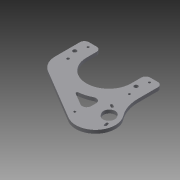
# Autodesk Inventor part: CAD:motor_plate
Saved by Autodesk Inventor 2015 (Build 190159000, 159)
## iProperties
Created: 2015-08-30
Material: Generic
Description: motor mount plate
Document SubType Name: Modeling
Designer: francis
Density: 1 g/cm^3
Appearance: Default
Part Category: insert part category here and press enter to fill value
Author: francis
Autodesk Inventor part; units mm, degrees
ref_plane "YZ Plane" through (0, 0, 0) normal (1, 0, 0) x (0, 1, 0)
ref_plane "XZ Plane" through (0, 0, 0) normal (0, 1, 0) x (-1, 0, 0)
ref_plane "XY Plane" through (0, 0, 0) normal (0, 0, 1) x (1, 0, 0)
sketch "Sketch1" plane through (0, 0, 0) normal (0, 0, 1) x (1, 0, 0)
  circle A0 centre (-18.2965, -47.165) radius 1.2295 construction
  circle A1 centre (-6.0724, -26.0926) radius 1.2295 construction
  circle A2 centre (5.6859, -42.8853) radius 1.2295 construction
  circle A3 centre (-0.1932, -34.489) radius 6 construction
  circle A4 centre (-7.5, -9) radius 1.621 construction
  circle A5 centre (-10.5, 0) radius 2.067 construction
  circle A6 centre (-7.5, 9) radius 1.621 construction
  circle A7 centre (-35, 0) radius 4 construction
  circle A8 centre (-62.5, 9) radius 1.621 construction
  line L0 (-55, -16) -> (-55, 16) construction
  circle A9 centre (-65.5, 0) radius 2.067 construction
  circle A10 centre (-62.5, -9) radius 1.621 construction
  circle A11 centre (-65.5, 0) radius 2.067 construction
  circle A12 centre (-62.5, 9) radius 1.7295 construction
  circle A13 centre (-62.5, -9) radius 1.7295 construction
  line L1 (-70, 13.1624) -> (-55, 13.1624) construction
  line L2 (-70, -13.1624) -> (-70, 13.1624) construction
  line L3 (-55, -13.1624) -> (-70, -13.1624) construction
  line L4 (-55, 13.1624) -> (-55, -13.1624) construction
  circle A14 centre (-10.5, 0) radius 2.067 construction
  circle A15 centre (-7.5, -9) radius 1.621 construction
  circle A16 centre (-7.5, 9) radius 1.621 construction
  line L5 (-15, 13.1624) -> (0, 13.1624) construction
  line L6 (-15, -13.1624) -> (-15, 13.1624) construction
  line L7 (0, -13.1624) -> (-15, -13.1624) construction
  line L8 (0, 13.1624) -> (0, -13.1624) construction
  arc A17 (4.363, -44.1343) -> (4.0127, -42.1709) centre (-18.2965, -47.165) ccw
  arc A18 (7.3366, -43.7366) -> (6.9402, -41.5156) centre (-18.2965, -47.165) ccw
  arc A19 (-5.9734, -27.9093) -> (-7.6985, -26.9086) centre (-18.2965, -47.165) ccw
  arc A20 (-4.3563, -25.3825) -> (-6.3078, -24.2504) centre (-18.2965, -47.165) ccw
  arc A21 (-4.9287, -38.6488) -> (-5.7218, -37.5161) centre (-18.2965, -47.165) ccw
  arc A22 (5.6137, -31.9325) -> (4.1951, -29.9066) centre (-18.2965, -47.165) ccw
  arc A23 (-5.1648, -26.6459) -> (-7.0032, -25.5795) centre (-18.2965, -47.165) ccw construction
  arc A24 (0.3425, -35.2907) -> (-0.7634, -33.7114) centre (-18.2965, -47.165) ccw construction
  arc A25 (5.8498, -43.9354) -> (5.4764, -41.8432) centre (-18.2965, -47.165) ccw construction
  arc A26 (6.9402, -41.5156) -> (4.0127, -42.1709) centre (5.4764, -41.8432) ccw
  arc A27 (4.363, -44.1343) -> (7.3366, -43.7366) centre (5.8498, -43.9354) ccw
  arc A28 (-4.9287, -38.6488) -> (5.6137, -31.9325) centre (0.3425, -35.2907) ccw
  arc A29 (4.1951, -29.9066) -> (-5.7218, -37.5161) centre (-0.7634, -33.7114) ccw
  arc A30 (-5.9734, -27.9093) -> (-4.3563, -25.3825) centre (-5.1648, -26.6459) ccw
  arc A31 (-6.3078, -24.2504) -> (-7.6985, -26.9086) centre (-7.0032, -25.5795) ccw
  circle A32 centre (-18.2965, -47.165) radius 1.5
  circle A33 centre (-7.5, -9) radius 2
  circle A34 centre (-7.5, 9) radius 2
  circle A35 centre (-10.5, 0) radius 2.5
  circle A36 centre (-62.5, 9) radius 2
  circle A37 centre (-65.5, 0) radius 2.5
  circle A38 centre (-62.5, -9) radius 2
  circle A39 centre (-7.3444, -39.4963) radius 17.7 construction
  arc A40 (-16.3879, -54.7116) -> (6.7463, -28.7846) centre (-7.3444, -39.4963) ccw
  arc A41 (0, -8.7624) -> (6.7463, -28.7846) centre (33.0845, -8.7624) ccw
  line L9 (0, -8.7624) -> (0, 9.1624)
  line L10 (-11, 13.1624) -> (-4, 13.1624)
  line L11 (-15, 9.1624) -> (-15, 0)
  line L12 (-55, 0) -> (-55, 9.1624)
  line L13 (-66, 13.1624) -> (-59, 13.1624)
  line L14 (-70, 9.1624) -> (-70, -13.1624)
  arc A42 (-55, 0) -> (-15, 0) centre (-35, 0) ccw
  arc A43 (-66, 13.1624) -> (-70, 9.1624) centre (-66, 9.1624) ccw
  arc A44 (-55, 9.1624) -> (-59, 13.1624) centre (-59, 9.1624) ccw
  arc A45 (-11, 13.1624) -> (-15, 9.1624) centre (-11, 9.1624) ccw
  arc A46 (0, 9.1624) -> (-4, 13.1624) centre (-4, 9.1624) ccw
  line L15 (-61.6755, -27.7942) -> (-16.3879, -54.7116)
  arc A47 (-70, -13.1624) -> (-61.6755, -27.7942) centre (-52.9789, -13.1624) ccw
  arc A48 (-35.0864, -30.8138) -> (-21.0883, -27.4948) centre (-35, 0) ccw
  line L16 (-35.0864, -30.8138) -> (-21.3261, -38.9925)
  line L17 (-15.2824, -31.0639) -> (-15.2824, -35.554)
  arc A49 (-15.2824, -31.0639) -> (-21.0883, -27.4948) centre (-19.2824, -31.0639) ccw
  arc A50 (-21.3261, -38.9925) -> (-15.2824, -35.554) centre (-19.2824, -35.554) ccw
  point P0 (0, 0)
  point P1 (-15.2824, -23.6794)
  dimension "d0" = 3
  dimension "d1" = 5
  dimension "d2" = 5
  dimension "d3" = 5
  dimension "d4" = 12.5
  dimension "d5" = 3
  dimension "d6" = 4
  dimension "d7" = 4
  dimension "d8" = 5
  dimension "d9" = 4
  dimension "d10" = 5
  dimension "d11" = 4
  dimension "d12" = 4
  dimension "d15" = 4
  constraints: 61 point on circle, 33 centre point, 29 tangent, 23 coincident, 20 end point, 10 point on line, 7 equal radius, 4 collinear, 2 midpoint, 1 perpendicular, 1 vertical
  measures "d0" radial gap between concentric circles of A18 A17
  measures "d4" radial gap between concentric circles of A22 A21
  measures "d5" diameter of A32
  measures "d6" diameter of A33
  measures "d7" diameter of A34
  measures "d8" diameter of A35
  measures "d9" diameter of A36
  measures "d10" diameter of A37
  measures "d11" diameter of A38
  measures "d12" radius of A43
  measures "d15" radius of A49
extrude "Extrusion1" add sketch "Sketch1" along normal blind 3
sketch "Sketch2" plane through (0, 0, 3) normal (0, 0, 1) x (1, 0, 0)
  arc A0 (4.1951, -29.9066) -> (-5.7218, -37.5161) centre (-0.7634, -33.7114) ccw projected
  arc A1 (5.6137, -31.9325) -> (4.1951, -29.9066) centre (-18.2965, -47.165) ccw projected
  arc A2 (-4.9287, -38.6488) -> (5.6137, -31.9325) centre (0.3425, -35.2907) ccw projected
  arc A3 (-4.9287, -38.6488) -> (-5.7218, -37.5161) centre (-18.2965, -47.165) ccw projected
  arc A4 (-35.0864, -30.8138) -> (-21.0883, -27.4948) centre (-35, 0) ccw projected
  arc A5 (-15.2824, -31.0639) -> (-21.0883, -27.4948) centre (-19.2824, -31.0639) ccw projected
  line L0 (-15.2824, -31.0639) -> (-15.2824, -35.554) projected
  arc A6 (-21.3261, -38.9925) -> (-15.2824, -35.554) centre (-19.2824, -35.554) ccw projected
  line L1 (-21.3261, -38.9925) -> (-35.0864, -30.8138) projected
  circle A7 centre (-65.5, 0) radius 2.5 projected
  circle A8 centre (-10.5, 0) radius 2.5 projected
  arc A9 (-6.3078, -24.2504) -> (-7.6985, -26.9086) centre (-7.0032, -25.5795) ccw projected
  arc A10 (-4.3563, -25.3825) -> (-6.3078, -24.2504) centre (-18.2965, -47.165) ccw projected
  arc A11 (-5.9734, -27.9093) -> (-4.3563, -25.3825) centre (-5.1648, -26.6459) ccw projected
  arc A12 (-5.9734, -27.9093) -> (-7.6985, -26.9086) centre (-18.2965, -47.165) ccw projected
  arc A13 (6.9402, -41.5156) -> (4.0127, -42.1709) centre (5.4764, -41.8432) ccw projected
  arc A14 (7.3366, -43.7366) -> (6.9402, -41.5156) centre (-18.2965, -47.165) ccw projected
  arc A15 (4.363, -44.1343) -> (7.3366, -43.7366) centre (5.8498, -43.9354) ccw projected
  arc A16 (4.363, -44.1343) -> (4.0127, -42.1709) centre (-18.2965, -47.165) ccw projected
  circle A17 centre (-62.5, -9) radius 2 projected
  circle A18 centre (-62.5, 9) radius 2 projected
  circle A19 centre (-7.5, 9) radius 2 projected
  circle A20 centre (-7.5, -9) radius 2 projected
  circle A21 centre (-18.2965, -47.165) radius 1.5 projected
  line L2 (-70, 9.1624) -> (-70, -13.1624) projected
  arc A22 (-70, -13.1624) -> (-61.6755, -27.7942) centre (-52.9789, -13.1624) ccw projected
  line L3 (-61.6755, -27.7942) -> (-16.3879, -54.7116) projected
  arc A23 (-16.3879, -54.7116) -> (6.7463, -28.7846) centre (-7.3444, -39.4963) ccw projected
  arc A24 (0, -8.7624) -> (6.7463, -28.7846) centre (33.0845, -8.7624) ccw projected
  line L4 (0, -8.7624) -> (0, 9.1624) projected
  arc A25 (0, 9.1624) -> (-4, 13.1624) centre (-4, 9.1624) ccw projected
  line L5 (-4, 13.1624) -> (-11, 13.1624) projected
  arc A26 (-11, 13.1624) -> (-15, 9.1624) centre (-11, 9.1624) ccw projected
  line L6 (-15, 9.1624) -> (-15, 0) projected
  arc A27 (-55, 0) -> (-15, 0) centre (-35, 0) ccw projected
  line L7 (-55, 0) -> (-55, 9.1624) projected
  arc A28 (-55, 9.1624) -> (-59, 13.1624) centre (-59, 9.1624) ccw projected
  line L8 (-59, 13.1624) -> (-66, 13.1624) projected
  arc A29 (-66, 13.1624) -> (-70, 9.1624) centre (-66, 9.1624) ccw projected
  circle A30 centre (-62.5, 9) radius 1
  circle A31 centre (-65.5, 0) radius 1.75
  circle A32 centre (-62.5, -9) radius 2 projected
  circle A33 centre (-62.5, -9) radius 1.1893
  circle A34 centre (-62.5, 9) radius 2
  circle A35 centre (-65.5, 0) radius 2.5
  circle A36 centre (-18.2965, -47.165) radius 1
  circle A37 centre (-7.5, -9) radius 1
  circle A38 centre (-7.5, 9) radius 1
  circle A39 centre (-10.5, 0) radius 1.75
  arc A40 (3.4017, -30.5154) -> (-4.9285, -36.9074) centre (-0.7634, -33.7114) ccw
  arc A41 (4.7703, -32.4698) -> (3.4017, -30.5154) centre (-18.2965, -47.165) ccw
  arc A42 (-4.0853, -38.1115) -> (4.7703, -32.4698) centre (0.3425, -35.2907) ccw
  arc A43 (-4.0853, -38.1115) -> (-4.9285, -36.9074) centre (-18.2965, -47.165) ccw
  arc A44 (6.4523, -41.6248) -> (4.5006, -42.0617) centre (5.4764, -41.8432) ccw
  arc A45 (6.841, -43.8029) -> (6.4523, -41.6248) centre (-18.2965, -47.165) ccw
  arc A46 (4.8586, -44.068) -> (6.841, -43.8029) centre (5.8498, -43.9354) ccw
  arc A47 (4.8586, -44.068) -> (4.5006, -42.0617) centre (-18.2965, -47.165) ccw
  arc A48 (-4.6258, -25.8036) -> (-6.5396, -24.6934) centre (-18.2965, -47.165) ccw
  arc A49 (-6.5396, -24.6934) -> (-7.4667, -26.4655) centre (-7.0032, -25.5795) ccw
  arc A50 (-5.7039, -27.4882) -> (-7.4667, -26.4655) centre (-18.2965, -47.165) ccw
  arc A51 (-5.7039, -27.4882) -> (-4.6258, -25.8036) centre (-5.1648, -26.6459) ccw
  point P0 (0, 0)
  dimension "d16" = 3.5
  dimension "d17" = 2
  dimension "d20" = 2
  dimension "d21" = 2
  dimension "d22" = 2
  dimension "d23" = 3.5
  dimension "d25" = 1
  dimension "d26" = 0.5
  dimension "d27" = 0.5
  constraints: 24 point on circle, 21 centre point, 9 coincident, 2 concentric, 9 other
  measures "d16" diameter of A31
  measures "d17" diameter of A30
  measures "d20" diameter of A36
  measures "d21" diameter of A37
  measures "d22" diameter of A38
  measures "d23" diameter of A39
  measures "d25" radial gap between concentric circles of A3 A43
  measures "d26" radial gap between concentric circles of A16 A47
  measures "d27" radial gap between concentric circles of A11 A51
extrude "Extrusion2" add sketch "Sketch2" against normal up to surface (3 mm away) contours A1 A2 A3 A0 | A7 | A8 | A10 A11 A12 A9 | A14 A15 A16 A13 | A17 | A18 | A19 | A20 | A21
fillet "Fillet1" radius 1 1 edges at (-35.0864, -30.8138, 1.5)
body "Solid1"
